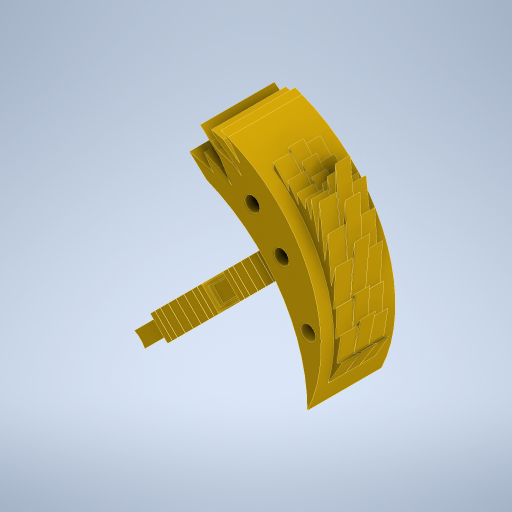
# Autodesk Inventor part: Sythic of death
Saved by Autodesk Inventor 2023 (Build 270158030, 158C)
## iProperties
Created: 2024-05-17
Part Number: Sythic of death
Material: Generic
Document SubType Name: Modeling
Designer: wa229389
Density: 1 g/cm^3
Appearance: Gold
Author: wa229389
Autodesk Inventor part; units mm, degrees
ref_plane "YZ Plane" through (0, 0, 0) normal (1, 0, 0) x (0, 1, 0)
ref_plane "XZ Plane" through (0, 0, 0) normal (0, 1, 0) x (-1, 0, 0)
ref_plane "XY Plane" through (0, 0, 0) normal (0, 0, 1) x (1, 0, 0)
sketch "Sketch1" plane through (0, 0, 0) normal (0, 0, 1) x (1, 0, 0)
  arc A0 (657.0224, 195.8578) -> (381, 871.015) centre (210.614, 407.3554) ccw
  arc A1 (0, 0) -> (-35.921, 35.921) centre (-68.7605, -32.8395) ccw
  arc A2 (657.0224, 195.8578) -> (538.8154, 538.8154) centre (109.2607, 198.9111) ccw
  arc A3 (538.8154, 538.8154) -> (312.567, 707.555) centre (109.2607, 198.9111) ccw
  line L0 (312.567, 707.555) -> (253.8263, 761.687)
  line L1 (253.8263, 761.687) -> (336.723, 740.9077)
  line L2 (336.723, 740.9077) -> (303.6642, 784.7667)
  line L3 (303.6642, 784.7667) -> (353.1824, 762.8372)
  line L4 (353.1824, 762.8372) -> (397.9516, 734.621)
  line L5 (397.9516, 734.621) -> (357.5022, 797.4238)
  line L6 (357.5022, 797.4238) -> (336.723, 816.5726)
  line L7 (336.723, 816.5726) -> (290.5396, 859.1325)
  line L8 (290.5396, 859.1325) -> (328.4233, 829.2334)
  line L9 (328.4233, 829.2334) -> (353.208, 813.6126)
  line L10 (353.208, 813.6126) -> (397.9516, 800.2092)
  line L11 (397.9516, 800.2092) -> (432.1943, 778.6274)
  line L12 (432.1943, 778.6274) -> (420.1035, 797.4)
  line L13 (420.1035, 797.4) -> (367.6772, 833.0167)
  line L14 (367.6772, 833.0167) -> (336.723, 854.0459)
  line L15 (336.723, 854.0459) -> (329.6193, 865.0752)
  line L16 (329.6193, 865.0752) -> (353.208, 859.5606)
  line L17 (353.208, 859.5606) -> (370.3802, 855.546)
  line L18 (370.3802, 855.546) -> (412.0838, 822.6321)
  arc A4 (412.0838, 822.6321) -> (426.1489, 815.2083) centre (439.2305, 857.0285) ccw
  line L19 (426.1489, 815.2083) -> (395.4249, 855.9696)
  line L20 (395.4249, 855.9696) -> (361.7941, 878.8173)
  line L21 (361.7941, 878.8173) -> (385.2896, 869.4161)
  line L22 (655.3893, 241.2865) -> (648.6444, 269.628)
  line L23 (648.6444, 269.628) -> (642.9643, 253.4448)
  line L24 (642.9643, 253.4448) -> (635.5109, 297.8183)
  line L25 (635.5109, 297.8183) -> (630.8434, 284.5201)
  line L26 (630.8434, 284.5201) -> (630.2587, 329.0869)
  line L27 (630.2587, 329.0869) -> (624.0209, 328.0391)
  line L28 (624.0209, 328.0391) -> (622.7423, 339.9309)
  line L29 (622.7423, 339.9309) -> (623.9241, 373.5002)
  line L30 (623.9241, 373.5002) -> (616.6657, 358.096)
  line L31 (616.6657, 358.096) -> (617.6828, 386.9845)
  line L32 (617.6828, 386.9845) -> (607.0555, 377.4058)
  line L33 (607.0555, 377.4058) -> (603.8352, 407.3554)
  line L34 (603.8352, 407.3554) -> (590.7177, 395.5322)
  line L35 (590.7177, 395.5322) -> (601.1213, 432.5947)
  line L36 (601.1213, 432.5947) -> (580.4296, 433.3232)
  line L37 (580.4296, 433.3232) -> (586.537, 455.0809)
  line L38 (586.537, 455.0809) -> (576.1096, 458.0079)
  line L39 (576.1096, 458.0079) -> (572.5425, 491.1816)
  line L40 (648.6444, 269.628) -> (639.2376, 223.3161)
  line L41 (639.2376, 223.3161) -> (652.0169, 232.7189)
  line L42 (652.0169, 232.7189) -> (655.3893, 209.4688)
  line L43 (655.3893, 209.4688) -> (656.7578, 216.206)
  line L44 (685.0008, 269.628) -> (745.3829, 365.7981)
  line L45 (745.3829, 365.7981) -> (715.1918, 343.584)
  line L46 (715.1918, 343.584) -> (737.8389, 455.0809)
  line L47 (737.8389, 455.0809) -> (711.0653, 412.4388)
  line L48 (711.0653, 412.4388) -> (718.709, 521.2073)
  line L49 (718.709, 521.2073) -> (703.7925, 497.4499)
  line L50 (703.7925, 497.4499) -> (718.709, 675.0559)
  line L51 (718.709, 675.0559) -> (695.8288, 562.411)
  line L52 (695.8288, 562.411) -> (685.0008, 781.9926)
  line L53 (685.0008, 781.9926) -> (674.0025, 625.4904)
  line L54 (674.0025, 625.4904) -> (652.0169, 874.1167)
  line L55 (652.0169, 874.1167) -> (652.0169, 672.2018)
  line L56 (652.0169, 672.2018) -> (623.9241, 822.6321)
  line L57 (623.9241, 822.6321) -> (627.1331, 724.6951)
  line L58 (627.1331, 724.6951) -> (607.0555, 793.3736)
  line L59 (607.0555, 793.3736) -> (608.5613, 747.417)
  line L60 (608.5613, 747.417) -> (570.6928, 793.3736)
  line L61 (570.6928, 793.3736) -> (584.1278, 747.417)
  line L62 (584.1278, 747.417) -> (536.9031, 822.6321)
  line L63 (536.9031, 822.6321) -> (552.174, 770.3953)
  line L64 (552.174, 770.3953) -> (491.9097, 843.5313)
  line L65 (491.9097, 843.5313) -> (498.3862, 808.8511)
  line L66 (461.1148, 618.7334) -> (468.7813, 594.2872)
  line L67 (468.7813, 594.2872) -> (441.9757, 629.85)
  line L68 (441.9757, 629.85) -> (435.2528, 615.3387)
  line L69 (435.2528, 615.3387) -> (404.3643, 656.3183)
  line L70 (404.3643, 656.3183) -> (399.7123, 644.7663)
  line L71 (399.7123, 644.7663) -> (379.6074, 671.4392)
  line L72 (379.6074, 671.4392) -> (379.6074, 650.5257)
  line L73 (379.6074, 650.5257) -> (360.9815, 676.7947)
  line L74 (360.9815, 676.7947) -> (360.9815, 657.0569)
  line L75 (360.9815, 657.0569) -> (333.9377, 695.1979)
  line L76 (333.9377, 695.1979) -> (333.9377, 677.9664)
  line L77 (333.9377, 677.9664) -> (322.1263, 703.6292)
  circle A5 centre (568.2701, 606.5103) radius 25.4
  circle A6 centre (660.1158, 427.8863) radius 25.4
  circle A7 centre (468.7813, 713.7542) radius 25.4
  line L78 (554.1402, 589.2909) -> (554.6884, 586.9874)
  line L79 (554.6884, 586.9874) -> (550.9222, 594.2872)
  line L80 (550.9222, 594.2872) -> (551.5556, 590.6373)
  line L81 (551.5556, 590.6373) -> (546.8438, 600.6195)
  line L82 (546.8438, 600.6195) -> (545.9401, 596.5603)
  line L83 (545.9401, 596.5603) -> (547.6534, 610.7875)
  line L84 (547.6534, 610.7875) -> (544.616, 606.5103)
  line L85 (544.616, 606.5103) -> (549.1997, 615.9474)
  line L86 (549.1997, 615.9474) -> (546.1347, 614.5006)
  line L87 (546.1347, 614.5006) -> (555.9763, 620.8393)
  line L88 (555.9763, 620.8393) -> (551.3449, 620.8393)
  line L89 (551.3449, 620.8393) -> (561.018, 625.4904)
  line L90 (561.018, 625.4904) -> (555.4345, 626.1628)
  line L91 (555.4345, 626.1628) -> (564.5477, 627.7443)
  line L92 (564.5477, 627.7443) -> (560.94, 629.4966)
  line L93 (560.94, 629.4966) -> (570.6503, 628.3273)
  line L94 (570.6503, 628.3273) -> (568.7801, 630.3713)
  line L95 (568.7801, 630.3713) -> (576.5881, 626.5788)
  line L96 (576.5881, 626.5788) -> (575.1435, 629.5831)
  line L97 (575.1435, 629.5831) -> (580.4296, 623.8057)
  line L98 (580.4296, 623.8057) -> (580.8265, 627.1018)
  line L99 (580.8265, 627.1018) -> (585.2391, 618.5491)
  line L100 (585.2391, 618.5491) -> (585.7943, 623.1597)
  line L101 (585.7943, 623.1597) -> (588.6754, 613.3044)
  line L102 (588.6754, 613.3044) -> (589.4967, 616.9937)
  line L103 (589.4967, 616.9937) -> (590.7532, 606.197)
  line L104 (589.9393, 598.8123) -> (591.911, 600.1832)
  line L105 (591.911, 600.1832) -> (586.898, 593.8315)
  line L106 (586.898, 593.8315) -> (589.9393, 594.2872)
  line L107 (589.9393, 594.2872) -> (582.5929, 589.5556)
  line L108 (582.5929, 589.5556) -> (585.5167, 589.8803)
  line L109 (585.5167, 589.8803) -> (579.3126, 587.4429)
  line L110 (579.3126, 587.4429) -> (582.7981, 585.8451)
  line L111 (582.7981, 585.8451) -> (575.5147, 585.9508)
  line L112 (575.5147, 585.9508) -> (578.7729, 584.7506)
  line L113 (578.7729, 584.7506) -> (572.0376, 584.5848)
  line L114 (572.0376, 584.5848) -> (574.5392, 583.6633)
  line L115 (554.1402, 589.2909) -> (560.5154, 583.8658)
  line L116 (560.5154, 583.8658) -> (559.6608, 585.8451)
  line L117 (559.6608, 585.8451) -> (568.2701, 582.803)
  line L118 (568.2701, 582.803) -> (564.9645, 584.9319)
  arc A8 (564.9645, 584.9319) -> (564.9645, 584.9319) centre (566.2593, 586.9423) ccw
  line L119 (564.9645, 584.9319) -> (574.5392, 583.6633)
  line L120 (590.7532, 606.197) -> (592.3845, 610.274)
  line L121 (592.3845, 610.274) -> (589.9393, 598.8123)
  circle A9 centre (468.7813, 713.7542) radius 25.4
  line L122 (454.6514, 696.5348) -> (455.1996, 694.2313)
  line L123 (455.1996, 694.2313) -> (451.4335, 701.5311)
  line L124 (451.4335, 701.5311) -> (452.0669, 697.8812)
  line L125 (452.0669, 697.8812) -> (447.355, 707.8634)
  line L126 (447.355, 707.8634) -> (446.4514, 703.8042)
  line L127 (446.4514, 703.8042) -> (448.1647, 718.0313)
  line L128 (448.1647, 718.0313) -> (445.1272, 713.7542)
  line L129 (445.1272, 713.7542) -> (449.7109, 723.1912)
  line L130 (449.7109, 723.1912) -> (446.6459, 721.7445)
  line L131 (446.6459, 721.7445) -> (456.4876, 728.0832)
  line L132 (456.4876, 728.0832) -> (451.8562, 728.0832)
  line L133 (451.8562, 728.0832) -> (461.5292, 732.7343)
  line L134 (461.5292, 732.7343) -> (455.9458, 733.4067)
  line L135 (455.9458, 733.4067) -> (465.0589, 734.9882)
  line L136 (465.0589, 734.9882) -> (461.4512, 736.7405)
  line L137 (461.4512, 736.7405) -> (471.1615, 735.5712)
  line L138 (471.1615, 735.5712) -> (469.2914, 737.6152)
  line L139 (469.2914, 737.6152) -> (477.0994, 733.8227)
  line L140 (477.0994, 733.8227) -> (475.6548, 736.827)
  line L141 (475.6548, 736.827) -> (480.9408, 731.0496)
  line L142 (480.9408, 731.0496) -> (481.3377, 734.3457)
  line L143 (481.3377, 734.3457) -> (485.7503, 725.793)
  line L144 (485.7503, 725.793) -> (486.3055, 730.4036)
  line L145 (486.3055, 730.4036) -> (489.1866, 720.5483)
  line L146 (489.1866, 720.5483) -> (490.0079, 724.2376)
  line L147 (490.0079, 724.2376) -> (491.2644, 713.4409)
  line L148 (490.4505, 706.0562) -> (492.4222, 707.4271)
  line L149 (492.4222, 707.4271) -> (487.4092, 701.0754)
  line L150 (487.4092, 701.0754) -> (490.4505, 701.5311)
  line L151 (490.4505, 701.5311) -> (483.1041, 696.7995)
  line L152 (483.1041, 696.7995) -> (486.0279, 697.1242)
  line L153 (486.0279, 697.1242) -> (479.8238, 694.6868)
  line L154 (479.8238, 694.6868) -> (483.3093, 693.089)
  line L155 (483.3093, 693.089) -> (476.0259, 693.1947)
  line L156 (476.0259, 693.1947) -> (479.2842, 691.9945)
  line L157 (479.2842, 691.9945) -> (472.5489, 691.8287)
  line L158 (472.5489, 691.8287) -> (475.0505, 690.9072)
  line L159 (454.6514, 696.5348) -> (461.0267, 691.1097)
  line L160 (461.0267, 691.1097) -> (460.172, 693.089)
  line L161 (460.172, 693.089) -> (468.7813, 690.0469)
  line L162 (468.7813, 690.0469) -> (465.4758, 692.1758)
  arc A10 (465.4758, 692.1758) -> (465.4758, 692.1758) centre (466.7706, 694.1862) ccw
  line L163 (465.4758, 692.1758) -> (475.0505, 690.9072)
  line L164 (491.2644, 713.4409) -> (492.8957, 717.5178)
  line L165 (492.8957, 717.5178) -> (490.4505, 706.0562)
  circle A11 centre (660.1158, 427.8863) radius 25.4
  line L166 (645.9859, 410.6668) -> (646.5341, 408.3633)
  line L167 (646.5341, 408.3633) -> (642.7679, 415.6632)
  line L168 (642.7679, 415.6632) -> (643.4013, 412.0133)
  line L169 (643.4013, 412.0133) -> (638.6895, 421.9955)
  line L170 (638.6895, 421.9955) -> (637.7859, 417.9362)
  line L171 (637.7859, 417.9362) -> (639.4991, 432.1634)
  line L172 (639.4991, 432.1634) -> (636.4617, 427.8863)
  line L173 (636.4617, 427.8863) -> (641.0454, 437.3233)
  line L174 (641.0454, 437.3233) -> (637.9804, 435.8766)
  line L175 (637.9804, 435.8766) -> (647.822, 442.2153)
  line L176 (647.822, 442.2153) -> (643.1907, 442.2153)
  line L177 (643.1907, 442.2153) -> (652.8637, 446.8664)
  line L178 (652.8637, 446.8664) -> (647.2803, 447.5388)
  line L179 (647.2803, 447.5388) -> (656.3934, 449.1203)
  line L180 (656.3934, 449.1203) -> (652.7857, 450.8726)
  line L181 (652.7857, 450.8726) -> (662.496, 449.7033)
  line L182 (662.496, 449.7033) -> (660.6258, 451.7472)
  line L183 (660.6258, 451.7472) -> (668.4338, 447.9548)
  line L184 (668.4338, 447.9548) -> (666.9892, 450.9591)
  line L185 (666.9892, 450.9591) -> (672.2753, 445.1817)
  line L186 (672.2753, 445.1817) -> (672.6722, 448.4778)
  line L187 (672.6722, 448.4778) -> (677.0848, 439.9251)
  line L188 (677.0848, 439.9251) -> (677.64, 444.5356)
  line L189 (677.64, 444.5356) -> (680.5211, 434.6803)
  line L190 (680.5211, 434.6803) -> (681.3424, 438.3697)
  line L191 (681.3424, 438.3697) -> (682.5989, 427.573)
  line L192 (681.785, 420.1882) -> (683.7567, 421.5592)
  line L193 (683.7567, 421.5592) -> (678.7437, 415.2075)
  line L194 (678.7437, 415.2075) -> (681.785, 415.6632)
  line L195 (681.785, 415.6632) -> (674.4386, 410.9316)
  line L196 (674.4386, 410.9316) -> (677.3624, 411.2562)
  line L197 (677.3624, 411.2562) -> (671.1583, 408.8189)
  line L198 (671.1583, 408.8189) -> (674.6438, 407.2211)
  line L199 (674.6438, 407.2211) -> (667.3604, 407.3268)
  line L200 (667.3604, 407.3268) -> (670.6186, 406.1266)
  line L201 (670.6186, 406.1266) -> (663.8833, 405.9608)
  line L202 (663.8833, 405.9608) -> (666.3849, 405.0393)
  line L203 (645.9859, 410.6668) -> (652.3612, 405.2418)
  line L204 (652.3612, 405.2418) -> (651.5065, 407.2211)
  line L205 (651.5065, 407.2211) -> (660.1158, 404.179)
  line L206 (660.1158, 404.179) -> (656.8102, 406.3079)
  arc A12 (656.8102, 406.3079) -> (656.8102, 406.3079) centre (658.105, 408.3183) ccw
  line L207 (656.8102, 406.3079) -> (666.3849, 405.0393)
  line L208 (682.5989, 427.573) -> (684.2302, 431.6499)
  line L209 (684.2302, 431.6499) -> (681.785, 420.1882)
  line L210 (216.784, 311.9747) -> (46.0158, 141.2065)
  line L211 (46.0158, 136.7164) -> (100.7954, 81.9368)
  line L212 (221.2741, 311.9747) -> (276.0537, 257.1951)
  line L213 (105.2855, 81.9368) -> (276.0537, 252.705)
  line L214 (548.9493, 525.6006) -> (550.4897, 527.141)
  line L215 (-35.921, 35.921) -> (55.4451, 127.2871)
  line L216 (0, 0) -> (91.3661, 91.3661)
  line L217 (465.1788, 560.3695) -> (294.4106, 389.6014)
  line L218 (294.4106, 385.1112) -> (349.1902, 330.3317)
  line L219 (469.6689, 560.3695) -> (524.4485, 505.59)
  line L220 (353.6803, 330.3317) -> (524.4485, 501.0998)
  line L221 (230.7034, 302.5454) -> (303.8399, 375.682)
  line L222 (479.0982, 550.9403) -> (505.3945, 577.2365)
  line L223 (266.6244, 266.6244) -> (339.7609, 339.7609)
  line L224 (515.0192, 515.0192) -> (538.8154, 538.8154)
  arc A13 (46.0158, 141.2065) -> (46.0158, 136.7164) centre (48.2609, 138.9614) ccw
  arc A14 (100.7954, 81.9368) -> (105.2855, 81.9368) centre (103.0404, 84.1819) ccw
  arc A15 (276.0537, 252.705) -> (276.0537, 257.1951) centre (273.8086, 254.9501) ccw
  arc A16 (221.2741, 311.9747) -> (216.784, 311.9747) centre (219.029, 309.7296) ccw
  arc A17 (294.4106, 389.6014) -> (294.4106, 385.1112) centre (296.6557, 387.3563) ccw
  arc A18 (349.1902, 330.3317) -> (353.6803, 330.3317) centre (351.4353, 332.5767) ccw
  arc A19 (524.4485, 501.0998) -> (524.4485, 505.59) centre (522.2034, 503.3449) ccw
  arc A20 (469.6689, 560.3695) -> (465.1788, 560.3695) centre (467.4239, 558.1245) ccw
  dimension "d0" = 762
  dimension "d4" = 76.2
  dimension "d5" = 50.8
  dimension "d6" = 50.8
  dimension "d7" = 50.8
  dimension "d8" = 50.8
  dimension "d9" = 50.8
  dimension "d11" = 3.175
  constraints: 450 end point, 61 parallel, 52 point on line, 44 point on circle, 27 perpendicular, 21 centre point, 20 tangent, 8 equal radius, 3 horizontal, 2 vertical
  measures "d0" distance of L224.end L216.start
  measures "d4" radius of A1
  measures "d5" diameter of A5
  measures "d6" diameter of A6
  measures "d7" diameter of A7
  measures "d8" diameter of A9
  measures "d9" diameter of A11
  measures "d11" radius of A13
extrude "Extrusion1" add sketch "Sketch1" along normal mid plane 254 contours A2 A3 L0 L1 L2 L3 L4 L5 L6 L7 L8 L9 L10 L11 L12 L13 L14 L15 L16 L17 L18 A4 L19 L20 L21 A0
extrude "Extrusion2" add sketch "Sketch1" along normal mid plane 101.6 contours L219 A19 L220 A18 L218 A17 L217 A20 | L212 A15 L213 A14 L211 A13 L210 A16
extrude "Extrusion3" add sketch "Sketch1" along normal mid plane 50.8 contours L224 L219 L222 A3 | L223 L212 L221 L218 | L216 A1 L215 L211
extrude "Extrusion4" add sketch "Sketch1" along normal mid plane 50.8 contours A0 L65 L64 L63 L62 L61 L60 L59 L58 L57 L56 L55 L54 L53 L52 L51 L50 L49 L48 L47 L46 L45 L44 | L43 L42 L41 L40 L22 A2 | L22 L23 L24 L25 L26 L27 L28 L29 L30 L31 L32 L33 L34 L35 L36 L37 L38 L39 A2 | L66 L67 L68 L69 L70 L71 L72 L73 L74 L75 L76 L77 A3
extrude "Extrusion5" add sketch "Sketch1" along normal mid plane 152.4 contours A5 | A6 | A7 | L119 A8 | L163 A10 | L207 A12 picked at (566.1403, 584.7188) picked at (466.3064, 692.0084) picked at (657.986, 406.0948)
sketch "Sketch2" plane through (0, 0, 50.8) normal (0, 0, 1) x (1, 0, 0)
  line L0 (294.4106, 389.6014) -> (465.1788, 560.3695) projected
  line L1 (379.7947, 474.9854) -> (439.0644, 415.7157)
  line L2 (353.6803, 330.3317) -> (524.4485, 501.0998) projected
  line L3 (216.784, 311.9747) -> (46.0158, 141.2065) projected
  line L4 (131.3999, 226.5906) -> (190.6696, 167.3209)
  line L5 (105.2855, 81.9368) -> (276.0537, 252.705) projected
  line L6 (325.9132, 421.1039) -> (385.1829, 361.8342)
  line L7 (433.6763, 528.867) -> (492.9459, 469.5973)
  line L8 (185.2814, 280.4721) -> (244.5511, 221.2024)
  line L9 (77.5183, 172.7091) -> (136.788, 113.4394)
  line L10 (307.9527, 403.1434) -> (367.2224, 343.8737)
  line L11 (203.2419, 298.4326) -> (262.5116, 239.163)
  line L12 (59.5578, 154.7485) -> (118.8275, 95.4789)
  line L13 (104.4591, 199.6498) -> (163.7288, 140.3801)
  line L14 (158.3407, 253.5314) -> (217.6103, 194.2617)
  line L15 (406.7355, 501.9262) -> (466.0052, 442.6565)
  line L16 (352.854, 448.0447) -> (412.1236, 388.775)
  line L17 (451.6368, 546.8275) -> (510.9065, 487.5578)
  line L18 (452.5348, 547.7255) -> (511.8045, 488.4558)
  line L19 (434.5743, 529.765) -> (493.844, 470.4953)
  line L20 (407.6335, 502.8242) -> (466.9032, 443.5545)
  line L21 (380.6927, 475.8835) -> (439.9624, 416.6138)
  line L22 (353.752, 448.9427) -> (413.0217, 389.673)
  line L23 (326.8112, 422.0019) -> (386.0809, 362.7322)
  line L24 (308.8507, 404.0414) -> (368.1204, 344.7717)
  line L25 (204.14, 299.3307) -> (263.4096, 240.061)
  line L26 (186.1794, 281.3702) -> (245.4491, 222.1005)
  line L27 (159.2387, 254.4294) -> (218.5084, 195.1597)
  line L28 (132.2979, 227.4886) -> (191.5676, 168.2189)
  line L29 (60.4559, 155.6466) -> (119.7256, 96.3769)
  line L30 (78.4164, 173.6071) -> (137.6861, 114.3374)
  line L31 (105.3571, 200.5479) -> (164.6268, 141.2782)
  point P0 (0, 0)
  dimension "d22" = 76.2
  dimension "d23" = 76.2
  dimension "d24" = 76.2
  dimension "d25" = 76.2
  dimension "d26" = 25.4
  dimension "d27" = 25.4
  dimension "d28" = 25.4
  dimension "d29" = 38.1
  dimension "d30" = 38.1
  dimension "d31" = 38.1
  dimension "d32" = 38.1
  dimension "d33" = 25.4
  dimension "d34" = 1.27
  dimension "d35" = 1.27
  dimension "d36" = 1.27
  dimension "d37" = 1.27
  dimension "d39" = 1.27
  dimension "d40" = 1.27
  dimension "d41" = 1.27
  dimension "d42" = 1.27
  dimension "d43" = 1.27
  dimension "d44" = 1.27
  dimension "d45" = 1.27
  dimension "d46" = 1.27
  dimension "d47" = 1.27
  dimension "d48" = 1.27
  constraints: 56 end point, 26 parallel, 4 midpoint
  measures "d22" distance between parallel lines of L1 L6
  measures "d23" distance between parallel lines of L1 L7
  measures "d24" distance between parallel lines of L4 L8
  measures "d25" distance between parallel lines of L4 L9
  measures "d26" distance between parallel lines of L6 L10
  measures "d27" distance between parallel lines of L8 L11
  measures "d28" distance between parallel lines of L9 L12
  measures "d29" distance between parallel lines of L4 L13
  measures "d30" distance between parallel lines of L4 L14
  measures "d31" distance between parallel lines of L1 L15
  measures "d32" distance between parallel lines of L1 L16
  measures "d33" distance between parallel lines of L7 L17
  measures "d34" distance between parallel lines of L17 L18
  measures "d35" distance between parallel lines of L7 L19
  measures "d36" distance between parallel lines of L15 L20
  measures "d37" distance between parallel lines of L1 L21
  measures "d39" distance between parallel lines of L16 L22
  measures "d40" distance between parallel lines of L6 L23
  measures "d41" distance between parallel lines of L10 L24
  measures "d42" distance between parallel lines of L11 L25
  measures "d43" distance between parallel lines of L8 L26
  measures "d44" distance between parallel lines of L14 L27
  measures "d45" distance between parallel lines of L4 L28
  measures "d46" distance between parallel lines of L12 L29
  measures "d47" distance between parallel lines of L9 L30
  measures "d48" distance between parallel lines of L13 L31
extrude "Extrusion6" cut sketch "Sketch2" against normal blind 101.6 contours L0 L24 L2 L10 | L0 L23 L2 L6 | L0 L22 L2 L16 | L0 L21 L2 L1 | L0 L20 L2 L15 | L0 L19 L2 L7 | L0 L18 L2 L17 | L25 L5 L11 L3 | L26 L5 L8 L3 | L27 L5 L14 L3 | L28 L5 L4 L3 | L31 L5 L13 L3 | L30 L5 L9 L3 | L29 L5 L12 L3
sketch "Sketch4" plane through (118.8275, 95.4789, -50.8) normal (0.7071068, 0.7071068, 0) x (-0.7071068, 0.7071068, 0)
  line L0 (83.82, 0) -> (83.82, 101.6) projected
  line L1 (0, 0) -> (3.175, 0) projected
  line L2 (83.82, 101.6) -> (0, 101.6)
  line L3 (0, 101.6) -> (0, 0)
  line L4 (0, 0) -> (83.82, 0)
  line L5 (83.82, 0) -> (83.82, 101.6)
  line L6 (12.7, 88.9) -> (71.12, 88.9)
  line L7 (71.12, 88.9) -> (71.12, 12.7)
  line L8 (71.12, 12.7) -> (12.7, 12.7)
  line L9 (12.7, 12.7) -> (12.7, 88.9)
  point P0 (16.51, 50.8)
  dimension "d78" = 12.7
  constraints: 16 end point, 4 parallel, 2 perpendicular, 1 horizontal, 3 other
  measures "d78" distance between parallel lines of L2 L6
extrude "Extrusion7" add sketch "Sketch4" along normal blind 228.6 and the other way blind 38.1 contours L6 L7 L8 L9
sketch "Sketch5" plane through (367.2224, 343.8737, -50.8) normal (0.7071068, 0.7071068, 0) x (-0.7071068, 0.7071068, 0)
  line L0 (12.7, 12.7) -> (71.12, 12.7)
  line L1 (71.12, 12.7) -> (71.12, 88.9)
  line L2 (71.12, 88.9) -> (12.7, 88.9)
  line L3 (12.7, 88.9) -> (12.7, 12.7)
  point P0 (16.51, 50.8)
  point P1 (83.82, 0)
  point P2 (0, 101.6)
  constraints: 8 end point, 2 parallel, 1 perpendicular
extrude "Extrusion8" add sketch "Sketch5" along normal blind 228.6 and the other way blind 25.4
sketch "Sketch6" plane through (0, 0, 25.4) normal (0, 0, 1) x (1, 0, 0)
  arc A0 (685.0008, 269.628) -> (498.3862, 808.8511) centre (210.614, 407.3554) ccw
  line L0 (498.3862, 808.8511) -> (498.3862, 830.422)
  line L1 (552.174, 770.3953) -> (491.9097, 843.5313) projected
  line L2 (498.3862, 830.422) -> (552.174, 770.3953)
  line L3 (552.174, 770.3953) -> (547.0654, 800.4086)
  line L4 (584.1278, 747.417) -> (570.6928, 793.3736) projected
  line L5 (547.0654, 800.4086) -> (584.1278, 747.417)
  line L6 (584.1278, 747.417) -> (578.7114, 779.2387)
  line L7 (570.6928, 793.3736) -> (608.5613, 747.417) projected
  line L8 (578.7114, 779.2387) -> (608.5613, 747.417)
  line L9 (608.5613, 747.417) -> (609.4142, 778.128)
  line L10 (627.1331, 724.6951) -> (607.0555, 793.3736) projected
  line L11 (609.4142, 778.128) -> (627.1331, 724.6951)
  line L12 (627.1331, 724.6951) -> (627.1331, 785.402)
  line L13 (652.0169, 874.1167) -> (652.0169, 672.2018) projected
  line L14 (627.1331, 785.402) -> (652.0169, 672.2018)
  line L15 (652.0169, 672.2018) -> (655.3327, 791.6008)
  line L16 (674.0025, 625.4904) -> (652.0169, 874.1167) projected
  line L17 (655.3327, 791.6008) -> (674.0025, 625.4904)
  line L18 (674.0025, 625.4904) -> (685.0008, 710.831)
  line L19 (685.0008, 781.9926) -> (695.8288, 562.411) projected
  line L20 (685.0008, 710.831) -> (695.8288, 562.411)
  line L21 (695.8288, 562.411) -> (711.2508, 625.4904)
  line L22 (718.709, 675.0559) -> (703.7925, 497.4499) projected
  line L23 (711.2508, 625.4904) -> (703.7925, 497.4499)
  line L24 (703.7925, 497.4499) -> (714.3689, 507.3709)
  line L25 (711.0653, 412.4388) -> (718.709, 521.2073) projected
  line L26 (714.3689, 507.3709) -> (711.0653, 412.4388)
  line L27 (711.0653, 412.4388) -> (729.6329, 434.3796)
  line L28 (737.8389, 455.0809) -> (715.1918, 343.584) projected
  line L29 (729.6329, 434.3796) -> (715.1918, 343.584)
  line L30 (715.1918, 343.584) -> (734.5719, 354.2749)
  arc A1 (685.0008, 269.628) -> (498.3862, 808.8511) centre (210.614, 407.3554) ccw projected
  line L31 (734.5719, 354.2749) -> (685.0008, 269.628)
  arc A2 (657.0224, 195.8578) -> (312.567, 707.555) centre (109.2607, 198.9111) ccw projected
  arc A3 (459.3156, 620.2348) -> (322.1263, 703.6292) centre (109.2607, 198.9111) ccw
  line L32 (322.1263, 703.6292) -> (332.542, 682.9582)
  line L33 (333.9377, 677.9664) -> (333.9377, 695.1979) projected
  line L34 (332.542, 682.9582) -> (333.9377, 695.1979)
  line L35 (333.9377, 695.1979) -> (357.9556, 666.221)
  line L36 (360.9815, 676.7947) -> (360.9815, 657.0569) projected
  line L37 (357.9556, 666.221) -> (360.9815, 676.7947)
  line L38 (360.9815, 676.7947) -> (376.7219, 657.8043)
  line L39 (379.6074, 671.4392) -> (379.6074, 650.5257) projected
  line L40 (376.7219, 657.8043) -> (379.6074, 671.4392)
  line L41 (379.6074, 671.4392) -> (398.1472, 651.6322)
  line L42 (435.2528, 615.3387) -> (404.3643, 656.3183) projected
  line L43 (398.1472, 651.6322) -> (404.3643, 656.3183)
  line L44 (404.3643, 656.3183) -> (434.2725, 620.2348)
  line L45 (434.2725, 620.2348) -> (441.9757, 629.85)
  line L46 (441.9757, 629.85) -> (463.2909, 604.1338)
  line L47 (461.1148, 618.7334) -> (468.7813, 594.2872) projected
  line L48 (463.2909, 604.1338) -> (461.1148, 618.7334)
  line L49 (656.7578, 216.206) -> (655.3893, 209.4688) projected
  line L50 (576.1096, 458.0079) -> (572.5425, 491.1816) projected
  arc A4 (656.7578, 216.206) -> (572.5425, 491.1816) centre (109.2607, 198.9111) ccw
  line L51 (572.5425, 491.1816) -> (577.6078, 459.9048)
  line L52 (580.4296, 433.3232) -> (601.1213, 432.5947) projected
  line L53 (582.5976, 435.0063) -> (601.1213, 432.5947)
  line L54 (601.1213, 432.5947) -> (595.0628, 403.3199)
  line L55 (603.8352, 407.3554) -> (607.0555, 377.4058) projected
  line L56 (595.0628, 403.3199) -> (603.8352, 407.3554)
  line L57 (586.537, 455.0809) -> (576.1096, 458.0079) projected
  line L58 (577.6078, 459.9048) -> (586.537, 455.0809)
  line L59 (586.537, 455.0809) -> (582.5976, 435.0063)
  line L60 (603.8352, 407.3554) -> (607.6671, 381.6468)
  line L61 (617.6828, 386.9845) -> (607.0555, 377.4058) projected
  line L62 (607.6671, 381.6468) -> (617.6828, 386.9845)
  line L63 (617.6828, 386.9845) -> (618.2736, 366.3785)
  line L64 (623.9241, 373.5002) -> (616.6657, 358.096) projected
  line L65 (618.2736, 366.3785) -> (623.9241, 373.5002)
  line L66 (623.9241, 373.5002) -> (625.5991, 330.414)
  line L67 (630.2587, 329.0869) -> (624.0209, 328.0391) projected
  line L68 (625.5991, 330.414) -> (630.2587, 329.0869)
  line L69 (630.2587, 329.0869) -> (632.0497, 292.767)
  line L70 (642.9643, 253.4448) -> (635.5109, 297.8183) projected
  line L71 (632.0497, 292.767) -> (635.5109, 297.8183)
  line L72 (635.5109, 297.8183) -> (643.0644, 263.4564)
  line L73 (639.2376, 223.3161) -> (648.6444, 269.628) projected
  line L74 (643.0644, 263.4564) -> (648.6444, 269.628)
  line L75 (648.6444, 269.628) -> (643.0644, 230.0243)
  line L76 (655.3893, 209.4688) -> (652.0169, 232.7189) projected
  line L77 (643.0644, 230.0243) -> (652.0169, 232.7189)
  line L78 (652.0169, 232.7189) -> (655.3893, 213.4517)
  line L79 (655.3893, 213.4517) -> (656.7578, 216.206)
  point P0 (0, 0)
  constraints: 108 end point, 8 point on circle, 6 parallel, 3 centre point, 2 perpendicular, 1 vertical
extrude "Extrusion9" add sketch "Sketch6" along normal blind 58.42 and the other way blind 101.6 contours A0 L0 L2 L3 L5 L6 L8 L9 L11 L12 L14 L15 L17 L18 L20 L21 L23 L24 L26 L27 L29 L30 L31 | L79 L78 L77 L75 L74 L72 L71 L69 L68 L66 L65 L63 L62 L60 L56 L54 L53 L59 L58 L51 A2 | L48 L46 L45 L44 L43 L41 L40 L38 L37 L35 L34 L32 A2
body "Solid1"
